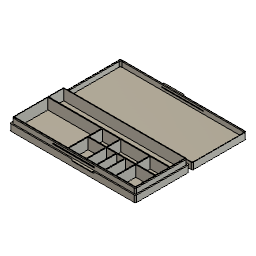
ywit_2025_box (Autodesk Fusion 360 design; units mm, degrees)
Autodesk Fusion 360 part; units mm, degrees
sketch "Sketch1" plane through (0, 0, 0) normal (0, 1, 0) x (1, 0, 0)
  line L0 (-85.9353, 37.5516) -> (129.0647, 37.5516)
  line L1 (129.0647, 37.5516) -> (129.0647, -52.4484)
  line L2 (129.0647, -52.4484) -> (-85.9353, -52.4484)
  line L3 (-85.9353, -52.4484) -> (-85.9353, 37.5516)
  dimension "d1" = 215
  dimension "d2" = 90
  constraint horizontal L0
  constraint vertical L1
  constraint horizontal L2
  constraint vertical L3
  measures "d1" distance of L0.start L0.end
  measures "d2" distance of L0.start L2.end
extrude "Extrude1" add sketch "Sketch1" along normal blind 21 makes body 1
shell "Shell1" thickness 2 removed faces 1 at (-14.2686, 21, 22.4484) on bodies 1
sketch "Sketch2" plane through (0, 2, 0) normal (0, 1, 0) x (-1, 0, 0)
  line L0 (83.9353, 50.4484) -> (-127.0647, 50.4484)
  line L1 (-127.0647, 50.4484) -> (-127.0647, -35.5516)
  line L2 (-127.0647, -35.5516) -> (83.9353, -35.5516)
  line L3 (83.9353, -35.5516) -> (83.9353, 50.4484)
  line L4 (83.9353, 50.4484) -> (-11.0647, 50.4484)
  line L5 (-11.0647, 50.4484) -> (-11.0647, -9.5516)
  line L6 (-11.0647, -9.5516) -> (83.9353, -9.5516)
  line L7 (83.9353, -9.5516) -> (83.9353, 50.4484)
  line L8 (-11.0647, 15.4484) -> (-127.0647, 15.4484)
  line L9 (-43.0647, 15.4484) -> (-43.0647, 50.4484)
  line L10 (-61.0647, 15.4484) -> (-61.0647, 50.4484)
  line L11 (-76.0647, 15.4484) -> (-76.0647, 50.4484)
  line L12 (-11.0647, -9.5516) -> (-127.0647, -9.5516)
  line L13 (-43.0647, -9.5516) -> (-43.0647, 15.4484)
  line L14 (-11.0647, -8.0516) -> (83.9353, -8.0516)
  line L15 (-11.0647, -8.0516) -> (-127.0647, -8.0516)
  line L16 (-11.0647, 16.9484) -> (-94.0647, 16.9484)
  line L17 (-9.5647, 50.4484) -> (-9.5647, -9.5516)
  line L18 (-41.5647, 15.4484) -> (-41.5647, 50.4484)
  line L19 (-41.5647, -9.5516) -> (-41.5647, 15.4484)
  line L20 (-59.5647, 15.4484) -> (-59.5647, 50.4484)
  line L21 (-74.5647, 15.4484) -> (-74.5647, 50.4484)
  line L22 (-94.0647, -9.5516) -> (-94.0647, 15.4484)
  line L23 (-94.0647, 15.4484) -> (-94.0647, 50.4484)
  line L24 (-92.5647, -9.5516) -> (-92.5647, 50.4484)
  line L25 (-94.0647, 16.9484) -> (-127.0647, 16.9484)
  dimension "d33" = 95
  dimension "d34" = 60
  dimension "d35" = 35
  dimension "d36" = 32
  dimension "d37" = 18
  dimension "d38" = 15
  dimension "d39" = 32
  dimension "d40" = 1.5
  dimension "d41" = 1.5
  dimension "d42" = -1.5
  dimension "d43" = 1.5
  dimension "d44" = 1.5
  dimension "d45" = 1.5
  dimension "d46" = 1.5
  dimension "d130" = 1.5
  dimension "d131" = 33
  constraint horizontal L4
  constraint vertical L5
  constraint horizontal L6
  constraint vertical L7
  constraint coincident L0.start L3.end
  constraint coincident L5 L8.start
  constraint coincident L1 L8.end
  constraint perpendicular L1 L8
  constraint coincident L8 L9.start
  constraint coincident L0 L9.end
  constraint perpendicular L0 L9
  constraint coincident L8 L10.start
  constraint coincident L0 L10.end
  constraint perpendicular L0 L10
  constraint coincident L8 L11.start
  constraint coincident L0 L11.end
  constraint perpendicular L0 L11
  constraint coincident L1 L12.end
  constraint perpendicular L1 L12
  constraint coincident L12 L13.start
  constraint perpendicular L12 L13
  constraint coincident L12 L22.start
  constraint coincident L8 L22.end
  constraint perpendicular L8 L22
  constraint coincident L0 L23.end
  constraint perpendicular L0 L23
  constraint coincident L12 L24.start
  constraint perpendicular L16 L24
  constraint coincident L16.end L23
  constraint coincident L1 L25.end
  constraint perpendicular L1 L25
  constraint coincident L0 L24.end
  measures "d33" distance of L0.start L4.end
  measures "d34" distance of L0.start L6.end
  measures "d35" distance of L0 L8
  measures "d36" distance of L5 L9
  measures "d37" distance of L9 L10
  measures "d38" distance of L10 L11
  measures "d39" distance of L5 L13
  measures "d130" distance of L22 L24
  measures "d131" distance of L1 L23
extrude "Extrude3" add sketch "Sketch2" along normal up to surface (19 mm away) contours L0 L4 L5 L14 L17 | L3 L6 L7 L14 L17 | L5 L6 L14 L17 | L0 L9 L16 L18 | L5 L8 L16 L18 | L5 L12 L15 L19 | L8 L9 L16 L18 | L12 L13 L15 L19 | L8 L13 L15 L19 | L0 L10 L16 L20 | L8 L9 L16 L20 | L12 L13 L15 L24 | L1 L12 L15 L22 | L8 L10 L16 L20 | L12 L15 L22 L24 | L8 L15 L22 L24 | L0 L11 L16 L21 | L8 L10 L16 L21 | L8 L11 L16 L24 | L8 L16 L23 L24 | L1 L8 L23 L25 | L8 L11 L16 L21 | L0 L16 L23 L24 bodies 1
fillet "Fillet1" radius 7 9 edges at (26.3147, 2, 50.4484) (51.3147, 2, 50.4484) (67.8147, 2, 50.4484) (84.3147, 2, 50.4484) (110.5647, 2, 50.4484) (67.8147, 2, 15.4484) (110.5647, 2, 15.4484) (26.3147, 2, 15.4484) (21.5647, 2, -9.5516) on bodies 1
sketch "Sketch4" plane through (0, 0, 0) normal (0, -1, 0) x (1, 0, 0)
  line L0 (129.0647, 52.4484) -> (-85.9353, 52.4484)
  line L1 (-85.9353, 52.4484) -> (-85.9353, -37.5516)
  line L2 (-85.9353, -37.5516) -> (129.0647, -37.5516)
  line L3 (129.0647, -37.5516) -> (129.0647, 52.4484)
  line L4 (-87.9353, -39.5516) -> (131.0647, -39.5516)
  line L5 (131.0647, -39.5516) -> (131.0647, 54.4484)
  line L6 (131.0647, 54.4484) -> (-87.9353, 54.4484)
  line L7 (-87.9353, 54.4484) -> (-87.9353, -39.5516)
  dimension "d30" = 2
extrude "Extrude4" add sketch "Sketch4" against normal blind 10.5 bodies 1
fillet "Fillet2" radius 2 4 edges at (-85.9353, 15.75, 52.4484) (129.0647, 15.75, 52.4484) (129.0647, 15.75, -37.5516) (-85.9353, 15.75, -37.5516) on bodies 1
extrude "Extrude13" add 1 faces at (-13.602, 10.5, -38.8849) along direction (0, 1, 0) blind 1 on bodies 1 bodies 1
sketch "Sketch6" plane through (0, 11.5, 0) normal (0, 1, 0) x (-1, 0, 0)
  arc A0 (-92.0647, 52.4484) -> (-94.0647, 50.4484) centre (-92.0647, 50.4484) ccw
  line L0 (-92.0647, 52.4484) -> (83.9353, 52.4484)
  arc A1 (85.9353, 50.4484) -> (83.9353, 52.4484) centre (83.9353, 50.4484) ccw
  line L1 (85.9353, 50.4484) -> (85.9353, -35.5516)
  arc A2 (83.9353, -37.5516) -> (85.9353, -35.5516) centre (83.9353, -35.5516) ccw
  line L2 (83.9353, -37.5516) -> (-92.0647, -37.5516)
  arc A3 (-94.0647, -35.5516) -> (-92.0647, -37.5516) centre (-92.0647, -35.5516) ccw
  line L3 (-94.0647, -35.5516) -> (-94.0647, 50.4484)
  line L4 (87.9353, -39.5516) -> (87.9353, 54.4484)
  line L5 (87.9353, 54.4484) -> (-96.0647, 54.4484)
  line L6 (-96.0647, 54.4484) -> (-96.0647, -39.5516)
  line L7 (-96.0647, -39.5516) -> (87.9353, -39.5516)
  arc A4 (-127.0647, 52.4484) -> (-129.0647, 50.4484) centre (-127.0647, 50.4484) ccw
  line L8 (-127.0647, 52.4484) -> (83.9353, 52.4484)
  arc A5 (85.9353, 50.4484) -> (83.9353, 52.4484) centre (83.9353, 50.4484) ccw
  line L9 (85.9353, 50.4484) -> (85.9353, -35.5516)
  arc A6 (83.9353, -37.5516) -> (85.9353, -35.5516) centre (83.9353, -35.5516) ccw
  line L10 (83.9353, -37.5516) -> (-127.0647, -37.5516)
  arc A7 (-129.0647, -35.5516) -> (-127.0647, -37.5516) centre (-127.0647, -35.5516) ccw
  line L11 (-129.0647, -35.5516) -> (-129.0647, 50.4484)
  line L12 (87.9353, -39.5516) -> (87.9353, 54.4484)
  line L13 (87.9353, 54.4484) -> (-131.0647, 54.4484)
  line L14 (-131.0647, 54.4484) -> (-131.0647, -39.5516)
  line L15 (-131.0647, -39.5516) -> (87.9353, -39.5516)
extrude "Extrude5" add sketch "Sketch6" along normal up to surface (11.5 mm away) separate body contours L0 A1 L1 A2 L2 L4 L5 L6 L7 L8 A5 L9 A6 L10 L12 L13 L15 | L6 A4 L8 L10 A7 L11 L13 L14 L15 makes body 2
sketch "Sketch7" plane through (0, 23, 0) normal (0, 1, 0) x (-1, 0, 0)
  line L0 (85.9353, 50.4484) -> (85.9353, -35.5516)
  arc A0 (83.9353, -37.5516) -> (85.9353, -35.5516) centre (83.9353, -35.5516) ccw
  line L1 (83.9353, -37.5516) -> (-127.0647, -37.5516)
  line L2 (-127.0647, 52.4484) -> (83.9353, 52.4484)
  arc A1 (85.9353, 50.4484) -> (83.9353, 52.4484) centre (83.9353, 50.4484) ccw
  line L3 (-131.0647, -39.5516) -> (87.9353, -39.5516)
  line L4 (87.9353, -39.5516) -> (87.9353, 54.4484)
  line L5 (87.9353, 54.4484) -> (-131.0647, 54.4484)
  arc A2 (-129.0647, -35.5516) -> (-127.0647, -37.5516) centre (-127.0647, -35.5516) ccw
  line L6 (-129.0647, -35.5516) -> (-129.0647, 50.4484)
  arc A3 (-127.0647, 52.4484) -> (-129.0647, 50.4484) centre (-127.0647, 50.4484) ccw
  line L7 (-131.0647, 54.4484) -> (-131.0647, -39.5516)
extrude "Extrude6" add sketch "Sketch7" against normal up to surface (2 mm away) contours L0 A0 L1 L2 A1 A2 L6 A3 bodies 2
move_face "OffsetFaces1" offset -0.4 8 faces at (56.7314, 14.6667, 52.4484) (-85.9263, 14.6667, 50.6385) (-85.9353, 17.8333, 21.7818) (-13.602, 14.6667, -37.5516) (-85.5645, 14.6667, -36.7117) (129.0647, 14.6667, -6.8849) (128.5122, 17.8333, 51.8286) (128.6938, 14.6667, -36.7117) on bodies 2
sketch "Sketch8" plane through (-85.9353, 0, 0) normal (-1, 0, 0) x (0, 0, 1)
  line L0 (-35.5516, 21) -> (-35.5516, 11.5)
  line L1 (50.4484, 11.5) -> (50.4484, 21)
  line L2 (50.4484, 21) -> (-35.5516, 21)
  line L3 (52.4484, 11.5) -> (52.4484, 21)
  line L4 (52.4484, 17.1) -> (52.4484, 15.4)
  line L5 (52.4484, 16.25) -> (50.4484, 16.25) construction
  line L6 (52.4484, 15.4) -> (53.0484, 16)
  line L7 (52.4484, 15.4) -> (53.1017, 15.4) construction
  line L8 (52.4484, 17.1) -> (53.0484, 16.5)
  line L9 (52.4484, 17.1) -> (53.0089, 17.1) construction
  line L10 (53.0484, 16.5) -> (53.0484, 16)
  line L11 (-35.5516, 11.5) -> (50.4484, 11.5)
  dimension "d58" = 1.7
  dimension "d61" = 45
  dimension "d62" = 45
  dimension "d126" = 0.6
  constraint coincident L3 L4.start
  constraint vertical L4
  constraint midpoint L3 L5.start
  constraint midpoint L1 L5.end
  constraint symmetric L4.start L4.end L5
  constraint horizontal L7
  constraint horizontal L9
  constraint vertical L10
  constraint coincident L8.end L10.start
  constraint coincident L6.end L10.end
  measures "d58" distance of L4.start L4.end
  measures "d61" angle of L6 L7
  measures "d62" angle of L8 L9
  measures "d126" distance of L5.start L10
extrude "Extrude7" add sketch "Sketch8" against normal blind 71.6667 from surface at -71.6667 contours L3 L4 L6 L8 L10 bodies 1
combine "Combine1" operation cut target body 2 tool bodies 1 keep tools
move_face "OffsetFaces2" offset -0.1 5 faces at (9.6202, 16.6333, 52.9151) (9.6202, 16.3333, 53.0484) (57.398, 16.3333, 52.9151) (-14.2686, 16.3333, 52.9151) (9.6202, 15.8667, 52.9151) on bodies 2
sketch "Sketch10" plane through (0, 0, 54.4484) normal (0, 0, 1) x (1, 0, 0)
  line L0 (-87.9353, 0) -> (131.0647, 0)
  line L1 (131.0647, 0) -> (131.0647, 11.5)
  line L2 (-87.9353, 11.5) -> (-87.9353, 0)
  line L3 (21.5647, 11.5) -> (21.5647, 0) construction
  line L4 (21.5647, 11.5) -> (57.398, 11.5)
  line L5 (57.398, 11.5) -> (57.398, 8.5)
  line L6 (57.398, 8.5) -> (21.5647, 8.5)
  line L7 (21.5647, 8.5) -> (21.5647, 11.5)
  line L8 (131.0647, 11.5) -> (-87.9353, 11.5)
  dimension "d68" = 35.8333
  dimension "d69" = 3
  constraint midpoint L0 L3.end
  constraint horizontal L4
  constraint vertical L5
  constraint horizontal L6
  constraint vertical L7
  constraint collinear L4 L8
  measures "d68" distance of L3.start L4.end
  measures "d69" distance of L4.end L5.end
extrude "Extrude8" add sketch "Sketch10" along normal blind 2 contours L4 L5 L6 L7 L8 bodies 1
chamfer "Chamfer1" distance 2 angle 45 1 edges at (39.4814, 8.5, 56.4484) on bodies 1
fillet "Fillet3" radius 1 4 edges at (21.5647, 10, 54.4484) (21.5647, 11, 56.4484) (57.398, 11, 56.4484) (57.398, 10, 54.4484) on bodies 1
sketch "Sketch11" plane through (0, 0, 54.4484) normal (0, 0, 1) x (1, 0, 0)
  line L0 (131.0647, 23) -> (-87.9353, 23)
  line L1 (-87.9353, 23) -> (-87.9353, 11.5)
  line L2 (21.5647, 23) -> (21.5647, 11.5) construction
  line L3 (21.5647, 11.5) -> (-14.2686, 11.5)
  line L4 (-14.2686, 11.5) -> (-14.2686, 14.5)
  line L5 (-14.2686, 14.5) -> (21.5647, 14.5)
  line L6 (21.5647, 14.5) -> (21.5647, 11.5)
  line L7 (-87.9353, 11.5) -> (131.0647, 11.5)
  line L8 (131.0647, 11.5) -> (131.0647, 23)
  dimension "d75" = 35.8333
  dimension "d76" = 3
  constraint midpoint L0 L2.start
  constraint horizontal L3
  constraint vertical L4
  constraint horizontal L5
  constraint vertical L6
  constraint vertical L2
  constraint collinear L3 L7
  measures "d75" distance of L2.end L3.end
  measures "d76" distance of L2.end L5.end
extrude "Extrude9" add sketch "Sketch11" along normal blind 2 contours L3 L4 L5 L6 L7 bodies 2
chamfer "Chamfer2" distance 2 angle 45 1 edges at (3.648, 14.5, 56.4484) on bodies 2
fillet "Fillet4" radius 1 4 edges at (-14.2686, 13, 54.4484) (-14.2686, 12, 56.4484) (21.5647, 13, 54.4484) (21.5647, 12, 56.4484) on bodies 2
sketch "Sketch12" plane through (-87.9353, 0, 0) normal (-1, 0, 0) x (0, 0, 1)
  line L0 (-39.5516, 0) -> (54.4484, 0)
  line L1 (54.4484, 0) -> (54.4484, 11.5)
  line L2 (-39.5516, 11.5) -> (-39.5516, 0)
  line L3 (-39.5516, 11.5) -> (-56.2713, 11.5) construction
  circle A0 centre (-42.0516, 11.5) radius 2
  line L4 (-43.4658, 10.0858) -> (-39.5516, 6.1716)
  line L5 (-43.4658, 10.0858) -> (-37.9615, 10.0858) construction
  line L6 (-40.2698, 12.4086) -> (-39.5516, 11)
  line L7 (54.4484, 11.5) -> (-39.5516, 11.5)
  dimension "d82" = 4
  dimension "d84" = 45
  dimension "d85" = 2.5
  dimension "d86" = 0.5
  constraint coincident L2.start L3.start
  constraint perpendicular L2 L3
  constraint coincident L3 A0.centre
  constraint horizontal L5
  constraint coincident A0 L4.start
  constraint coincident L2 L4.end
  constraint coincident A0 L6.start
  constraint coincident L2 L6.end
  constraint tangent A0 L4
  constraint tangent A0 L6
  measures "d82" diameter of A0
  measures "d84" angle of L4 L5
  measures "d85" distance of L2 A0.centre
  measures "d86" distance of L2.start L6.end
extrude "Extrude10" add sketch "Sketch12" against normal blind 3 from surface at -35.8333 contours L2 A0 L4 L6 | A0 bodies 1
pattern_linear "R-Pattern1" count 3 spacing 71.6667 along (1, 0, 0) of "Extrude10"
move_body "Move1" bodies 2 to x (1, 0, 0) y (0, -1, 0) z (0, 0, -1) at (0, 23, -79.1031)
move_body "Move2" bodies 2 to x (1, 0, 0) y (0, 1, 0) z (0, 0, 1) at (0, 0, -5)
sketch "Sketch13" plane through (-87.9353, 0, 0) normal (-1, 0, 0) x (0, 0, 1)
  line L0 (-138.5516, 0) -> (-44.5516, 0)
  line L1 (-44.5516, 0) -> (-44.5516, 11.5)
  line L2 (-138.5516, 11.5) -> (-138.5516, 0)
  line L3 (-43.4658, 10.0858) -> (-39.5516, 6.1716)
  line L4 (-39.5516, 6.1716) -> (-39.5516, 11)
  line L5 (-39.5516, 11) -> (-40.2698, 12.4086)
  arc A0 (-40.2698, 12.4086) -> (-43.4658, 10.0858) centre (-42.0516, 11.5) ccw
  circle A1 centre (-42.0516, 11.5) radius 2
  line L6 (-40.6397, 10.0835) -> (-44.5516, 6.1844)
  line L7 (-40.6397, 10.0835) -> (-35.1165, 10.0835) construction
  line L8 (-40.2698, 12.4086) -> (-43.8333, 12.4086) construction
  line L9 (-43.8333, 12.4086) -> (-44.5516, 11)
  line L10 (-44.5516, 11.5) -> (-138.5516, 11.5)
  dimension "d98" = 135.094
  constraint concentric A0 A1
  constraint coincident L5.end A1
  constraint horizontal L7
  constraint coincident A1 L6.start
  constraint tangent A1 L6
  constraint coincident L1 L6.end
  constraint horizontal L8
  constraint coincident L5.end A0.start
  constraint coincident A1 L8.end
  constraint coincident L1 L9.end
  constraint tangent A1 L9
  measures "d98" angle of L6 L7
extrude "Extrude11" add sketch "Sketch13" along normal blind 3 from surface at -35.6333 contours L1 L3 A0 A1 L6 L9 | L3 A1 L6 | A0 A1 bodies 2
ref_plane "WorkPlane1" through (-50.602, 9.8685, -41.9678) normal (1, 0, 0) x (0, 0, -1)
mirror "Mirror1" about plane through (-50.602, 9.8685, -41.9678) normal (1, 0, 0) of "Extrude11"
sketch "Sketch14" plane through (-48.902, 0, 0) normal (-1, 0, 0) x (0, 0, 1)
  line L0 (-43.8333, 12.4086) -> (-44.5516, 11)
  line L1 (-44.5516, 11) -> (-44.5516, 6.1844)
  line L2 (-44.5516, 6.1844) -> (-40.6397, 10.0835)
  arc A0 (-40.6397, 10.0835) -> (-43.8333, 12.4086) centre (-42.0516, 11.5) ccw
  circle A1 centre (-42.0516, 11.5) radius 1
  point P0 (-42.0516, 11.5)
  dimension "d108" = 2
  constraint concentric A0 A1
  constraint coincident P0 A0.centre
  measures "d108" diameter of A1
sphere "SpherePrimitive3" add diameter 2 placed x (0, 0, 1) y (0, 1, 0) z (-1, 0, 0) at (-48.902, 11.5, -42) bodies 2
mirror "Mirror2" about plane through (-50.602, 9.8685, -41.9678) normal (1, 0, 0) of "SpherePrimitive3"
pattern_linear "R-Pattern2" count 3 spacing 71.6667 along (1, 0, 0) of "Extrude11", "Mirror1", "SpherePrimitive3", "Mirror2"
combine "Combine2" operation cut target body 1 tool bodies 2 keep tools
move_face "OffsetFaces6" offset -0.2 6 faces at (94.1056, 10.6812, -41.5273) (91.3571, 12.3188, -42.4727) (19.6904, 10.6812, -42.4727) (22.439, 11.5, -42.9455) (-49.2277, 11.5, -42.9455) (-51.9762, 10.6812, -42.4727) on bodies 1
fillet "Fillet5" radius 2 8 edges at (-87.9353, 5.75, 54.4484) (-87.9353, 5.75, -39.5516) (131.0647, 5.75, -39.5516) (131.0647, 5.75, 54.4484) (-87.9353, 5.75, -44.5516) (-87.9353, 5.75, -138.5516) (131.0647, 5.75, -44.5516) (131.0647, 5.75, -138.5516) on bodies 1 2
chamfer "Chamfer3" distance 1 angle 45 16 edges at (21.5647, 21, 52.4484) (128.4789, 21, 51.8627) (129.0647, 21, 7.4484) (128.4789, 21, -36.9658) (21.5647, 21, -37.5516) (-85.3495, 21, -36.9658) (-85.9353, 21, 7.4484) (-85.3495, 21, 51.8627) (21.5647, 11.5, -136.9516) (-85.6324, 11.5, -136.2486) (-86.3353, 11.5, -91.5516) (-85.6324, 11.5, -46.8545) (21.5647, 11.5, -46.1516) (128.7617, 11.5, -46.8545) (129.4647, 11.5, -91.5516) (128.7617, 11.5, -136.2486) on bodies 1 2
move_body "Move5" [suppressed]
equation "d1 = box_length"
equation "d3 = box_depth"
equation "d31 = -box_depth / 2"
equation "d63 = -box_length / 3"
equation "d64 = -box_length / 3"
equation "box_length = 215 mm"
equation "d68 = box_length / 6"
equation "d75 = box_length / 6"
equation "d87 = -box_length / 6"
equation "d92 = -box_length / 3 * 2"
equation "d106 = box_length / 3 * 2"
equation "box_depth = 21 mm"
named bodies: "Base", "Lid"
